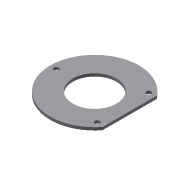
# Autodesk Inventor part: 00_Zeiss_Axiotech_Eyepiecemount
Saved by Autodesk Inventor 2019 (Build 230136000, 136)
## iProperties
Created: 2019-06-02
Part Number: 00_Zeiss_Axiotech_Eyepiecemount
Material: Generic
Document SubType Name: Modeling
Designer: diederichbenedict
Density: 1 g/cm^3
Appearance: Default
Author: diederichbenedict
Autodesk Inventor part; units mm, degrees
ref_plane "YZ Plane" through (0, 0, 0) normal (1, 0, 0) x (0, 1, 0)
ref_plane "XZ Plane" through (0, 0, 0) normal (0, 1, 0) x (-1, 0, 0)
ref_plane "XY Plane" through (0, 0, 0) normal (0, 0, 1) x (1, 0, 0)
sketch "Sketch1" plane through (0, 0, 0) normal (0, 1, 0) x (-1, 0, 0)
  circle A0 centre (0, 0) radius 1.75
  line L0 (0, 0) -> (-46.6476, -18) construction
  line L1 (-46.6476, -18) -> (-46.6476, 18) construction
  line L2 (-46.6476, 18) -> (0, 0) construction
  circle A1 centre (-46.6476, -18) radius 1.75 construction
  circle A2 centre (-46.6476, -18) radius 1.75
  circle A3 centre (-46.6476, 18) radius 1.75
  circle A4 centre (-34.2997, 0) radius 12.3479 construction
  arc A5 (0, 0) -> (-46.6476, 18) centre (-26.7967, 0) ccw construction
  arc A6 (-46.6476, 18) -> (-46.6476, -18) centre (-26.7967, 0) ccw construction
  arc A7 (-46.6476, -18) -> (0, 0) centre (-26.7967, 0) ccw construction
  circle A8 centre (-26.7967, 0) radius 31
  circle A9 centre (-26.7967, 0) radius 15.25
  line L3 (-51.2967, 18.9934) -> (-51.2967, -18.9934)
  dimension "d4" = 3.5
  dimension "d5" = 50
  dimension "d6" = 36
  dimension "d7" = 18
  dimension "d8" = 3.5
  dimension "d9" = 3.5
  dimension "d10" = 3.5
  dimension "d11" = 62
  dimension "d12" = 30.5
  dimension "d15" = 24.5
  constraints: 10 centre point, 9 point on circle, 8 end point, 6 coincident, 4 tangent, 2 vertical, 1 concentric, 1 point on line
  measures "d4" diameter of A0
  measures "d5" distance of L0.start L0.end
  measures "d6" distance of L0.end L1.end
  measures "d7" vertical distance of L0.start L0.end
  measures "d8" diameter of A1
  measures "d9" diameter of A2
  measures "d10" diameter of A3
  measures "d11" diameter of A8
  measures "d12" diameter of A9
  measures "d15" distance from line of A8.centre L3
extrude "Extrusion1" add sketch "Sketch1" along normal blind 2 contours A8 L3 picked at (-48.2134, 0)
body "Solid1"
